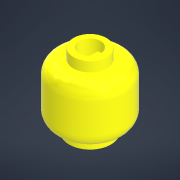
# Autodesk Inventor part: X02598_LEGOmini_Head_Y_Original_NoPara
Saved by Autodesk Inventor 2022 (Build 260153000, 153)
## iProperties
Created: 2014-07-02
Part Number: X02598_LEGOmini_Head_Y_Original_NoPara
Material: ABS Plastic
Document SubType Name: Modeling
Designer: D. Kohfeld
Mass: 0.601728 g
Surface Area: 5.85283 cm^2
Volume: 0.567668 cm^3
Density: 1.06 g/cm^3
Appearance: Yellow
Author: D. Kohfeld
Autodesk Inventor part; units mm, degrees
ref_plane "XZ Plane" through (0, 0, 0) normal (0, 1, 0) x (-1, 0, 0)
sketch "Sketch2" plane through (0, 0, 0) normal (0, 0, 1) x (1, 0, 0)
  line L0 (0, 4.1785) -> (1.6, 4.1785)
  line L1 (1.6, 4.1785) -> (1.6, 5.6785)
  line L2 (1.6, 5.6785) -> (2.5, 5.6785)
  line L3 (2.5, 5.6785) -> (2.5, 4.1785)
  line L4 (2.5, 4.1785) -> (3.2, 4.1785)
  arc A0 (5.2, 2.1785) -> (3.2, 4.1785) centre (3.2, 2.1785) ccw
  line L5 (5.2, 2.1785) -> (5.2, -2.1785)
  arc A1 (3.157, -4.2215) -> (5.2, -2.1785) centre (3.157, -2.1785) ccw
  line L6 (3.157, -4.2215) -> (3.157, -5.4215)
  line L7 (3.157, -5.4215) -> (2.5, -5.4215)
  line L8 (2.5, -5.4215) -> (2.5, 2.5785)
  line L9 (2.5, 2.5785) -> (0, 2.5785)
  line L10 (0, 2.5785) -> (0, 4.1785)
  point P0 (0, 0)
  point P1 (5.2, 0)
  dimension "d0" = 5
  dimension "d1" = 3.2
  dimension "d2" = 1.5
  dimension "d3" = 2
  dimension "d4" = 10.4
  dimension "d6" = 6.314
  dimension "d7" = 1.2
  dimension "d8" = 8
  dimension "d23" = 9.6
  constraints: 22 end point, 8 parallel, 4 point on circle, 3 tangent, 2 centre point, 2 horizontal alignment, 2 vertical alignment, 1 collinear, 1 horizontal, 1 midpoint, 1 perpendicular, 1 point on line
  measures "d0" diameter of L3 L10
  measures "d1" diameter of L1 L10
  measures "d2" distance from line of L2.end L4
  measures "d3" radius of A0
  measures "d4" diameter of L5 L10
  measures "d6" diameter of L6 L10
  measures "d7" distance from line of L7 L6.start
  measures "d8" distance from line of L7.end L9
  measures "d23" distance between parallel lines of L4 L7
revolve "Revolution1" add sketch "Sketch2" angle 360 about axis through (0, 2.5785, 0) along (0, 1, 0)
sketch "Sketch3" plane through (0, 4.1785, 0) normal (0, 1, 0) x (1, 0, 0)
  circle A0 centre (0, 0) radius 1.6 projected
  line L0 (-0.4, 1.5492) -> (-0.4, 0.2309)
  line L1 (-0.4, 0.2309) -> (-1.5416, -0.4282)
  line L2 (-1.1416, -1.121) -> (0, -0.4619)
  line L3 (0, -0.4619) -> (1.1416, -1.121)
  line L4 (1.5416, -0.4282) -> (0.4, 0.2309)
  line L5 (0.4, 0.2309) -> (0.4, 1.5492)
  dimension "d10" = 120
  dimension "d11" = 0.8
  constraints: 12 end point, 6 point on circle, 5 equal length, 3 parallel, 1 horizontal alignment, 1 vertical
  measures "d10" angle of L1 L0
  measures "d11" distance between parallel lines of L5 L0
extrude "Extrusion1" cut sketch "Sketch3" against normal through all contours A0 L4 L5 | L0 L1 A0 | A0 L2 L3
fillet "Fillet1" radius 0.1 2 edges at (-2.5, 5.6785, 0) (-3.157, -5.4215, 0)
ref_plane "Work Plane1" through (5.2, 0, 0) normal (1, 0, 0) x (0, 1, 0)
ref_plane "Work Plane2" through (0, 0, 5.2) normal (0, 0, 1) x (1, 0, 0)
sketch "草圖6" plane through (0, 0, 0) normal (0, 0, 1) x (1, 0, 0)
  line L0 (-4.1434, 3.1407) -> (-0.5207, 1.6675)
  arc A0 (-4.1434, 3.1407) -> (-0.5207, 1.6675) centre (-2.3321, 2.4041) ccw
  line L1 (0, 0) -> (0, 4.7535) construction
  line L2 (4.1434, 3.1407) -> (0.5207, 1.6675)
  arc A1 (0.5207, 1.6675) -> (4.1434, 3.1407) centre (2.3321, 2.4041) ccw
  line L3 (-3.0687, -0.588) -> (2.6358, -0.588)
  line L4 (2.5, -5.4215) -> (2.5, 2.5785) projected
  line L5 (2.6358, -0.588) -> (3.9705, -3.069)
  line L6 (3.9705, -3.069) -> (-3.887, -1.8285)
  line L7 (-3.887, -1.8285) -> (-3.0687, -0.588)
  point P0 (2.5, -2.8368)
  point P1 (2.5, -0.588)
  constraints: 14 end point, 4 point on circle, 3 symmetric about line, 2 centre point, 2 midpoint, 1 perpendicular, 1 vertical, 1 other
split_face "分割1"
split_face "分割2"
split_face "分割3"
ref_plane "工作平面3" through (0, -0.3215, 0) normal (0, 1, 0) x (-0.9999, 0, -0.015)
extrude "擠出2" add sketch "草圖6" along normal blind 5.5 separate body contours L0 A0 | A1 L4 L2 | L4 L6 L7 L3 | L4 A1 L2
body "Solid1"
